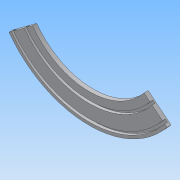
# Autodesk Inventor part: HOT Thermo bulb outline B
Saved by Autodesk Inventor 2013 (Build 170138000, 138)
## iProperties
Created: 2018-07-29
Part Number: HOT Thermo bulb outline B
Material: Generic
Document SubType Name: Modeling
Designer: Jeff Vyduna
Density: 1 g/cm^3
Author: Jeff Vyduna
Autodesk Inventor part; units mm, degrees
ref_plane "YZ Plane" through (0, 0, 0) normal (1, 0, 0) x (0, 1, 0)
ref_plane "XZ Plane" through (0, 0, 0) normal (0, 1, 0) x (-1, 0, 0)
ref_plane "XY Plane" through (0, 0, 0) normal (0, 0, 1) x (1, 0, 0)
ref_plane "Work Plane1" through (22.5184, 2.463, -18.3509) normal (0, 0, 1) x (0.9997722, -0.0213418, 0)
sketch "ThermoBulbBorder" plane through (22.5184, 2.463, -18.3509) normal (0, 0, 1) x (0.9997722, -0.0213418, 0)
  arc A0 (-447.455, -468.958) -> (162.145, -468.958) centre (-142.655, -774.8145) ccw
  arc A1 (-447.455, -468.958) -> (162.145, -468.958) centre (-142.655, -774.8145) ccw
  arc A2 (-383.955, -588.5959) -> (98.645, -588.5959) centre (-142.655, -774.8145) ccw
  line L0 (-447.455, -468.958) -> (-383.955, -468.958)
  line L1 (-383.955, -468.958) -> (-383.955, -588.5959)
  line L2 (162.145, -468.958) -> (98.645, -468.958)
  line L3 (98.645, -468.958) -> (98.645, -588.5959)
  line L4 (-383.955, -961.033) -> (-484.4967, -1038.6241)
  line L5 (98.645, -961.033) -> (199.1867, -1038.6241)
  arc A3 (-447.455, -468.958) -> (162.145, -468.958) centre (-142.655, -774.8145) ccw projected
  circle A4 centre (-142.655, -774.8145) radius 419.1 construction
  circle A5 centre (-142.655, -774.8145) radius 406.908 construction
  circle A6 centre (-142.655, -774.8145) radius 349.758 construction
  circle A7 centre (-142.655, -774.8145) radius 337.566 construction
  line L6 (98.645, -468.958) -> (98.645, -316.558) construction
  line L7 (-383.955, -468.958) -> (-383.955, -316.558) construction
  dimension "d0" = 609.6
  dimension "d5" = 63.5
  dimension "d6" = 63.5
  dimension "d7" = 838.2
  dimension "d8" = 12.192
  dimension "d9" = 12.192
  dimension "d10" = 57.15
  dimension "d11" = 32.766
  dimension "d12" = 152.4
  constraints: 16 end point, 12 point on circle, 7 centre point, 5 coincident, 2 concentric, 2 horizontal, 2 horizontal alignment, 2 line through centre, 2 parallel, 2 vertical, 2 vertical alignment, 1 collinear
  measures "d0" diameter of A2
  measures "d5" distance of L0.start L0.end
  measures "d6" distance of L2.start L2.end
  measures "d7" diameter of A4
  measures "d8" radial gap between concentric circles of A4 A5
  measures "d9" radial gap between concentric circles of A7 A6
  measures "d10" radial gap between concentric circles of A5 A6
  measures "d11" radial gap between concentric circles of A7 A2
  measures "d12" distance of L2.end L6.end
extrude "Extrusion2" add sketch "ThermoBulbBorder" along normal blind 18.034 contours L4 A2 L5 A0
sketch "Sketch2" plane through (22.5184, 2.463, -0.3169) normal (0, 0, 1) x (0.9997722, -0.0213418, 0)
  line L0 (-383.955, -961.033) -> (-484.4967, -1038.6241) projected
  arc A0 (-484.4967, -1038.6241) -> (199.1867, -1038.6241) centre (-142.655, -774.8145) ccw projected
  line L1 (199.1867, -1038.6241) -> (98.645, -961.033) projected
  arc A1 (-383.955, -961.033) -> (98.645, -961.033) centre (-142.655, -774.8145) ccw projected
  arc A2 (-409.8948, -981.0515) -> (124.5847, -981.0515) centre (-142.655, -774.8145) ccw
  arc A3 (-419.5468, -988.5003) -> (134.2367, -988.5003) centre (-142.655, -774.8145) ccw
  arc A4 (-464.7905, -1023.4163) -> (179.4805, -1023.4163) centre (-142.655, -774.8145) ccw
  arc A5 (-474.4425, -1030.865) -> (189.1325, -1030.865) centre (-142.655, -774.8145) ccw
  line L2 (-474.4425, -1030.865) -> (-464.7905, -1023.4163)
  line L3 (-419.5468, -988.5003) -> (-409.8948, -981.0515)
  line L4 (124.5847, -981.0515) -> (134.2367, -988.5003)
  line L5 (179.4805, -1023.4163) -> (189.1325, -1030.865)
  point P0 (-22.4607, -2.943)
  dimension "d15" = 12.192
  dimension "d17" = 12.7
  dimension "d18" = 57.15
  dimension "d19" = 12.192
  constraints: 8 end point, 8 point on circle, 8 point on line, 4 centre point, 4 collinear, 4 concentric
  measures "d15" radial gap between concentric circles of A4 A5
  measures "d17" radial gap between concentric circles of A0 A5
  measures "d18" radial gap between concentric circles of A4 A3
  measures "d19" radial gap between concentric circles of A2 A3
extrude "Extrusion3" cut sketch "Sketch2" against normal blind 12.7 contours A2 L1 A3 L0 | A4 L1 A5 L0
equation "\"d6\" = d5"
equation "\"d8\" = bRopeChannel"
equation "\"d9\" = bRopeChannel"
equation "\"d15\" = bRopeChannel"
equation "\"d19\" = bRopeChannel"
equation "\"bRopeChannel\" = 12.192"
body "Solid1"
